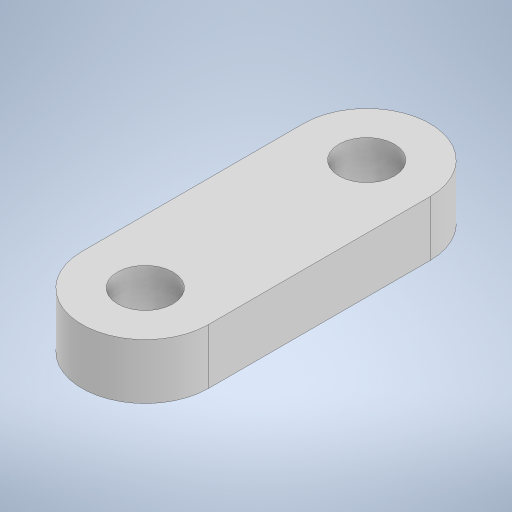
# Autodesk Inventor part: DIREcicon2opala
Saved by Autodesk Inventor 2023 (Build 270158000, 158)
## iProperties
Created: 2025-03-18
Part Number: DIREcicon2opala
Material: Genérico
Document SubType Name: Modeling
Designer: angel.dasilva
Density: 1 g/cm^3
Appearance: Valor por defecto
Author: angel.dasilva
Autodesk Inventor part; units mm, degrees
ref_plane "YZ Plane" through (0, 0, 0) normal (1, 0, 0) x (0, 1, 0)
ref_plane "XZ Plane" through (0, 0, 0) normal (0, 1, 0) x (-1, 0, 0)
ref_plane "XY Plane" through (0, 0, 0) normal (0, 0, 1) x (1, 0, 0)
sketch "Boceto1" plane through (0, 0, 0) normal (0, 1, 0) x (-1, 0, 0)
  arc A0 (-4, -16) -> (4, -16) centre (0, -16) ccw
  arc A1 (4, -2) -> (-4, -2) centre (0, -2) ccw
  line L0 (4, -2) -> (4, -16)
  line L1 (-4, -16) -> (-4, -2)
  line L2 (0, -4) -> (0, -2)
  circle A2 centre (0, -2) radius 1.75
  circle A3 centre (0, -16) radius 1.75
  point P0 (0, 0)
  dimension "d4" = 8
  dimension "d8" = 3.5
  dimension "d9" = 3.5
  constraints: 6 end point, 4 centre point, 4 point on circle, 2 coincident, 2 tangent, 1 vertical
  measures "d4" diameter of A1
  measures "d8" diameter of A2
  measures "d9" diameter of A3
extrude "Extrusión1" add sketch "Boceto1" along normal blind 3.5 contours L1 A1 L0 A0 | A2 | A3
extrude "Extrusión2" cut sketch "Boceto1" along normal blind 3.5 contours A2 | A3
